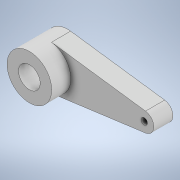
# Autodesk Inventor part: claw-t
Saved by Autodesk Inventor 2020 (Build 240168000, 168)
## iProperties
Created: 2020-11-06
Part Number: claw-t
Material: Generic
Document SubType Name: Modeling
Designer: alnwlsn
Density: 1 g/cm^3
Appearance: Default
Author: alnwlsn
Autodesk Inventor part; units mm, degrees
ref_plane "YZ Plane" through (0, 0, 0) normal (1, 0, 0) x (0, 1, 0)
ref_plane "XZ Plane" through (0, 0, 0) normal (0, 1, 0) x (-1, 0, 0)
ref_plane "XY Plane" through (0, 0, 0) normal (0, 0, 1) x (1, 0, 0)
sketch "Sketch1" plane through (0, 0, 0) normal (0, 0, 1) x (1, 0, 0)
  circle A0 centre (0, 0) radius 1.7
  circle A1 centre (0, 0) radius 3.5
  line L0 (0, 0) -> (15, 0) construction
  circle A2 centre (15, 0) radius 1.5
  circle A3 centre (15, 0) radius 0.5
  line L1 (0.4667, 3.4687) -> (15.2, 1.4866)
  line L2 (0.4667, -3.4687) -> (15.2, -1.4866)
  dimension "d0" = 3.4
  dimension "d1" = 7
  dimension "d2" = 3
  dimension "d3" = 1
  dimension "d4" = 15
  constraints: 6 end point, 4 centre point, 4 coincident, 4 point on circle, 4 tangent, 1 horizontal
  measures "d0" diameter of A0
  measures "d1" diameter of A1
  measures "d2" diameter of A2
  measures "d3" diameter of A3
  measures "d4" distance of L0.start L0.end
extrude "Extrusion1" add sketch "Sketch1" along normal blind 3
sketch "Sketch2" plane through (0, 0, 3) normal (0, 0, 1) x (1, 0, 0)
  line L0 (0.4667, -3.4687) -> (15.2, -1.4866) projected
  arc A0 (15.2, -1.4866) -> (15.2, 1.4866) centre (15, 0) ccw projected
  line L1 (15.2, 1.4866) -> (0.4667, 3.4687) projected
  arc A1 (0.4667, 3.4687) -> (0.4667, -3.4687) centre (0, 0) ccw projected
  circle A2 centre (15, 0) radius 0.5 projected
  circle A3 centre (0, 0) radius 1.7 projected
  arc A4 (0.4667, 3.4687) -> (0.4667, -3.4687) centre (0, 0) ccw projected
  circle A5 centre (0, 0) radius 3.5
  constraints: 1 coincident, 3 other
extrude "Extrusion2" add sketch "Sketch2" along normal blind 3 contours A1 A5
body "Solid1"
